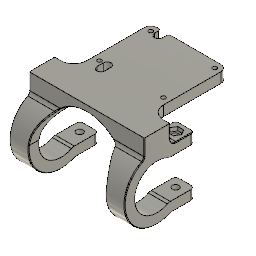
Screen Mount Assembly v8 (Autodesk Fusion 360 archive; units mm, degrees)
design "Mount"
Autodesk Fusion 360 part; units mm, degrees
note: some values were not read from the file. Set by a fixed rule: which face or edge a step refers to.
(part 1 of 2)
sketch "Sketch1" plane through (0, 0, -22.5) normal (0, 0, -1) x (1, 0, 0)
  circle A0 centre (-25, -20) radius 1.65
  circle A1 centre (25, 20) radius 1.65
  circle A2 centre (-25, 20) radius 1.65
  circle A3 centre (25, -20) radius 1.65
  circle A4 centre (25, 20) radius 5
  circle A5 centre (-25, 20) radius 5
  circle A6 centre (-25, -20) radius 5
  circle A7 centre (25, -20) radius 5
  line L0 (-25, -25) -> (25, -25)
  line L1 (30, -20) -> (30, 55)
  line L2 (30, 55) -> (-30, 55)
  line L3 (-30, 55) -> (-30, -20)
  line L4 (0, 0) -> (0, -45.9307) construction
  line L5 (0, 0) -> (62.0132, 0) construction
  dimension "d91" = 10
  dimension "d1" = 50
  dimension "d2" = 40
  dimension "d3" = 3.3
  dimension "d4" = 55
  constraint concentric A1 A4
  constraint concentric A2 A5
  constraint equal A4 A5
  constraint concentric A0 A6
  constraint concentric A3 A7
  constraint equal A4 A7
  constraint equal A4 A6
  constraint coincident A6 L0.start
  constraint coincident A7 L0.end
  constraint tangent A7 L0
  constraint tangent A6 L0
  constraint coincident A7 L1.start
  constraint tangent A7 L1
  constraint coincident A6 L3.end
  constraint tangent A6 L3
  constraint tangent A5 L3
  constraint tangent A4 L1
  constraint coincident L4.start L5.start
  constraint vertical L4
  constraint symmetric A0 A3 L4
  constraint symmetric A1 A2 L4
  constraint perpendicular L4 L5
  constraint symmetric A4 A7 L5
  constraint equal A1 A3
  constraint horizontal L2
  measures "d91" diameter of A4
  measures "d1" distance of A0.centre A3.centre
  measures "d2" distance of A1.centre A3.centre
  measures "d3" diameter of A3
  measures "d4" distance of L2 L5
extrude "Extrude1" add sketch "Sketch1" along normal blind 8 contours A4 | A5 | A6 A7 L0 L1 L2 L3 | A7 | A6
sketch "Sketch2" plane through (0, 0, -22.5) normal (0, 0, 1) x (-1, 0, 0)
  circle A0 centre (-25, -20) radius 1.65
  circle A1 centre (25, 20) radius 1.65
  circle A2 centre (25, -20) radius 1.65
  circle A3 centre (-25, 20) radius 1.65
  line L0 (30, -20) -> (30, 55)
  line L1 (30, 55) -> (-30, 55)
  line L2 (-30, 55) -> (-30, -20)
  arc A4 (-30, -20) -> (-25, -25) centre (-25, -20) ccw
  line L3 (-25, -25) -> (25, -25)
  arc A5 (25, -25) -> (30, -20) centre (25, -20) ccw
  line L4 (-30, 35) -> (-45, 35)
  line L5 (-45, 35) -> (-45, 55)
  line L6 (-45, 55) -> (-30, 55)
  line L7 (30, 55) -> (45, 55)
  line L8 (45, 55) -> (45, 35)
  line L9 (45, 35) -> (30, 35)
  line L10 (0, 55) -> (0, -10) construction
  dimension "d96" = 15
  dimension "d97" = 20
  constraint coincident L2 L4.start
  constraint perpendicular L2 L4
  constraint perpendicular L4 L5
  constraint coincident L1.end L2.start
  constraint perpendicular L2 L6
  constraint coincident L0.end L1.start
  constraint perpendicular L0 L7
  constraint perpendicular L7 L8
  constraint coincident L0 L9.end
  constraint perpendicular L0 L9
  constraint collinear L4 L9
  constraint midpoint L1 L10.start
  constraint perpendicular L1 L10
  constraint symmetric L5 L8 L10
  measures "d96" distance of L5.end L1.end
  measures "d97" distance of L4 L6
extrude "Extrude2" add sketch "Sketch2" against normal up to surface (8 mm away) contours L0 L7 L8 L9 | L2 L4 L5 L6
sketch "Sketch3" plane through (45, 0, 0) normal (1, 0, 0) x (0, 1, 0)
  line L0 (-55, -30.5) -> (-35, -30.5)
  line L1 (-35, -30.5) -> (-35, -22.5)
  line L2 (-35, -22.5) -> (-55, -22.5)
  line L3 (-55, -22.5) -> (-55, -30.5)
  circle A0 centre (-45, -60.5) radius 17.5
  circle A1 centre (-45, -60.5) radius 25.5
  line L4 (-35.9861, -45.5) -> (-15.5, -45.5)
  line L5 (-35.9861, -75.5) -> (-15.5, -75.5)
  line L6 (-27.5, -45.5) -> (-27.5, -75.5)
  line L7 (-45, -60.5) -> (22.9715, -60.5) construction
  line L8 (-55, -30.5) -> (-55, -37.0426)
  line L9 (-35, -30.5) -> (-35, -37.0426)
  line L10 (-45, -30.5) -> (-45, -60.5) construction
  line L11 (-33.9886, -37.5) -> (-15.5, -37.5)
  line L12 (-15.5, -37.5) -> (-15.5, -45.5)
  line L13 (-33.9886, -83.5) -> (-15.5, -83.5)
  line L14 (-15.5, -83.5) -> (-15.5, -75.5)
  dimension "d100" = 35
  dimension "d101" = 8
  dimension "d102" = 30
  dimension "d103" = 30
  dimension "d104" = 8
  dimension "d105" = 12
  constraint concentric A0 A1
  constraint coincident A0 L4.start
  constraint coincident A0 L5.start
  constraint horizontal L5
  constraint coincident L4 L6.start
  constraint coincident L5 L6.end
  constraint tangent A0 L6
  constraint vertical L6
  constraint coincident A0.centre A1.centre
  constraint horizontal L7
  constraint symmetric L4 L5 L7
  constraint coincident L0.start L3.end
  constraint coincident A1 L8.end
  constraint perpendicular L0 L8
  constraint coincident L0.end L1.start
  constraint coincident A1 L9.end
  constraint perpendicular L0 L9
  constraint midpoint L0 L10.start
  constraint perpendicular L0 L10
  constraint coincident A1 L11.start
  constraint parallel L4 L11
  constraint coincident A1 L13.start
  constraint perpendicular L12 L13
  constraint perpendicular L13 L14
  constraint collinear L12 L14
  constraint equal L12 L14
  measures "d100" diameter of A0 L7
  measures "d101" distance of A0 A1
  measures "d102" distance of L0 A0.centre
  measures "d103" distance of L4 L5
  measures "d104" distance of L4 L11
  measures "d105" distance of L6 L12
extrude "Extrude3" add sketch "Sketch3" against normal up to surface (90 mm away) contours L0 A1 L8 L9 | A0 A1 L4 L5 | A1 L5 L13 L14 | A1 L4 L11 L12
sketch "Sketch4" plane through (0, 0, -83.5) normal (0, 0, -1) x (1, 0, 0)
  circle A0 centre (37.5, 23) radius 2.65
  circle A1 centre (-37.5, 23) radius 2.65
  line L0 (0, 15.5) -> (0, 31.5) construction
  line L1 (-45, 33.9886) -> (-45, 15.5)
  line L2 (-45, 15.5) -> (45, 15.5)
  line L3 (45, 15.5) -> (45, 33.9886)
  line L4 (45, 33.9886) -> (-45, 33.9886)
  dimension "d109" = 5.3
  dimension "d25" = 7.5
  dimension "d26" = 7.5
  constraint symmetric A0 A1 L0
  constraint midpoint L0.start L2
  constraint perpendicular L0 L2
  measures "d109" diameter of A0
  measures "d25" distance of A0.centre L3
  measures "d26" distance of A0.centre L2
extrude "Extrude4" cut sketch "Sketch4" against normal up to surface (46 mm away) contours A0 | A1
sketch "Sketch7" plane through (0, 0, -37.5) normal (0, 0, 1) x (-1, 0, 0)
  circle A0 centre (-37.5, 23) radius 2.65
  circle A1 centre (37.5, 23) radius 2.65
  line L0 (45, 15.5) -> (45, 33.9886)
  line L1 (45, 33.9886) -> (-45, 33.9886)
  line L2 (-45, 33.9886) -> (-45, 15.5)
  line L3 (-45, 15.5) -> (45, 15.5)
  line L4 (35.1906, 27) -> (32.8812, 23)
  line L5 (32.8812, 23) -> (35.1906, 19)
  line L6 (35.1906, 19) -> (39.8094, 19)
  line L7 (39.8094, 19) -> (42.1188, 23)
  line L8 (42.1188, 23) -> (39.8094, 27)
  line L9 (39.8094, 27) -> (35.1906, 27)
  line L10 (-39.8094, 27) -> (-42.1188, 23)
  line L11 (-42.1188, 23) -> (-39.8094, 19)
  line L12 (-39.8094, 19) -> (-35.1906, 19)
  line L13 (-35.1906, 19) -> (-32.8812, 23)
  line L14 (-32.8812, 23) -> (-35.1906, 27)
  line L15 (-35.1906, 27) -> (-39.8094, 27)
  point P0 (37.5, 23)
  point P1 (-37.5, 23)
  dimension "d5" = 4
  constraint coincident P0 A1.centre
  constraint coincident A0.centre P1
  constraint horizontal L9
  constraint equal L9 L15
  constraint horizontal L15
  measures "d5" distance of P0 L9
extrude "Extrude5" cut sketch "Sketch7" against normal blind 3 contours L4 L5 L6 L7 L8 L9 | L10 L11 L12 L13 L14 L15
sketch "Sketch6" plane through (0, -55, 0) normal (0, -1, 0) x (1, 0, 0)
  line L0 (45, -22.5) -> (-45, -22.5)
  line L1 (-45, -22.5) -> (-45, -37.0426)
  line L2 (-45, -37.0426) -> (45, -37.0426)
  line L3 (45, -37.0426) -> (45, -22.5)
  line L4 (30, -30.5) -> (30, -91.7665)
  line L5 (45, -83.5) -> (45, -37.0426)
  line L6 (-30, -30.5) -> (-30, -95.0335)
  line L7 (-45, -80.5) -> (-45, -37.0426)
  line L8 (30, -30.5) -> (-30, -30.5)
  line L9 (-30, -30.5) -> (-25, -30.5)
  line L10 (-25, -30.5) -> (25, -30.5)
  line L11 (25, -30.5) -> (30, -30.5)
  line L12 (26.65, -30.5) -> (23.35, -30.5)
  line L13 (-23.35, -30.5) -> (-26.65, -30.5)
  line L14 (-23.35, -30.5) -> (-26.65, -30.5)
  line L15 (26.65, -30.5) -> (23.35, -30.5)
  arc A0 (30, -57.5) -> (-30, -57.5) centre (0, -57.5) ccw
  line L16 (40.15, -83.5) -> (34.85, -83.5)
  line L17 (-34.85, -83.5) -> (-40.15, -83.5)
  line L18 (-45, -83.5) -> (45, -83.5)
  line L19 (45, -83.5) -> (-45, -83.5)
  line L20 (-16.1649, -27.5) -> (17, -27.5) construction
  dimension "d31" = 3
  constraint coincident L2.end L3.start
  constraint coincident L1.end L2.start
  constraint perpendicular L2 L7
  constraint coincident L4.start L8.start
  constraint vertical L4
  constraint coincident L6.start L8.end
  constraint vertical L6
  constraint coincident L4 A0.start
  constraint tangent L6 A0
  constraint tangent L4 A0
  constraint coincident L6 A0.end
  constraint coincident L5.start L18.end
  constraint horizontal L20
  constraint tangent A0 L20
  measures "d31" distance of L8 L20
extrude "Extrude6" cut sketch "Sketch6" along normal blind 15.5 and the other way up to surface (39.5 mm away) contours L2 L4 L6 A0 L18 L19 | L2 L8 L10 A0 | L8 L10 A0
extrude "Extrude7" cut 1 faces at (-10, -41.3295, -83.5) along direction (0, 0, -1) blind 15
sketch "Sketch10" plane through (0, 0, -30.5) normal (0, 0, -1) x (1, 0, 0)
  line L0 (-13.0767, 35) -> (-30, 35)
  line L1 (-30, 35) -> (-30, -20)
  arc A0 (-30, -20) -> (-25, -25) centre (-25, -20) ccw
  line L2 (-25, -25) -> (25, -25)
  arc A1 (25, -25) -> (30, -20) centre (25, -20) ccw
  line L3 (30, -20) -> (30, 35)
  line L4 (30, 35) -> (13.0767, 35)
  circle A2 centre (-25, -20) radius 1.65
  circle A3 centre (25, 20) radius 1.65
  circle A4 centre (25, -20) radius 1.65
  circle A5 centre (-25, 20) radius 1.65
  line L5 (-13.0767, 15.5) -> (-13.0767, 35)
  line L6 (13.0767, 35) -> (13.0767, 15.5)
  line L7 (13.0767, 15.5) -> (-13.0767, 15.5)
extrude "Extrude9" cut sketch "Sketch10" along normal up to surface (53 mm away) contours L0 L1 A0 L2 A1 L3 L4 L5 L6 L7 | A2 | A3 | A4 | A5
fillet "Fillet1" radius 5 4 edges at (-37.5, -35.9861, -75.5) (37.5, -35.9861, -75.5) (-36.2477, -35.9861, -45.5) (36.2477, -35.9861, -45.5)
fillet "Fillet3" radius 5 4 edges at (37.5, -33.9886, -37.5) (-37.5, -33.9886, -37.5) (37.5, -35, -37.0426) (-37.5, -35, -37.0426)
fillet "Fillet3" radius 3 2 edges at (37.5, -33.9886, -83.5) (-37.5, -33.9886, -83.5)
fillet "Fillet3" radius 3 3 edges at (33.4715, -55, -37.0426) (-33.4715, -55, -37.0426) (33.4715, -55, -37.0426)
fillet "Fillet2" radius 5 2 edges at (-21.5383, -35, -30.5) (21.5383, -35, -30.5)
fillet "Fillet2" radius 10 2 edges at (-30, -35, -26.5) (30, -35, -26.5)
fillet "Fillet5" radius 3 6 edges at (-45, -15.5, -79.5) (-30, -15.5, -79.5) (45, -15.5, -79.5) (30, -15.5, -79.5) (45, -15.5, -41.5) (-45, -15.5, -41.5)
fillet "Fillet5" radius 3 2 edges at (-30, -15.5, -41.5) (30, -15.5, -41.5)
fillet "Fillet7" radius 2 4 edges at (-30, -35, -40.4953) (-30, -34.9421, -34.7412) (30, -34.9421, -34.7412) (30, -35, -40.4953)
fillet "Fillet8" radius 0.5 47 edges at (45, -55, -28.8188) (45, -55.4402, -36.702) (45, -67.9856, -71.5414) (45, -33.9557, -83.5665) (45, -25.9137, -83.5) (44.1213, -16.3787, -83.5) (37.5, -15.5, -83.5) (30.8787, -16.3787, -83.5) (30, -25.9137, -83.5) (30, -33.9557, -83.5665) (30, -60.0925, -81.054) (27.5466, -65.7069, -45.6182) (21.5129, -55.3759, -36.5909) (0, -55, -27.5) (-21.5129, -55.3759, -36.5909) (-27.5466, -65.7069, -45.6182) (-30, -60.0925, -81.054) (-30, -33.9557, -83.5665) (-30, -25.9137, -83.5) (-30.8787, -16.3787, -83.5) (-37.5, -15.5, -83.5) (-44.1213, -16.3787, -83.5) (-45, -25.9137, -83.5) (-45, -33.9557, -83.5665) (-45, -67.9856, -71.5414) (-45, -55.4402, -36.702) (-45, -55, -28.8188) (45, -35, -27.5) (45, -33.5355, -36.0355) (45, -24.25, -37.5) (44.1213, -16.3787, -37.5) (37.5, -15.5, -37.5) (30.8787, -16.3787, -37.5) (30, -24.25, -37.5) (30, -31.5811, -37.2434) (29.9254, -33.5435, -36.0277) (29.027, -34.6, -34.4596) (-45, -35, -27.5) (-45, -33.5355, -36.0355) (-45, -24.25, -37.5) (-44.1213, -16.3787, -37.5) (-37.5, -15.5, -37.5) (-30.8787, -16.3787, -37.5) (-30, -24.25, -37.5) (-30, -31.5811, -37.2434) (-29.9254, -33.5435, -36.0277) (-29.0637, -34.5848, -34.4949)
sketch "Sketch8" plane through (0, 0, -22.5) normal (0, 0, 1) x (-1, 0, 0)
  line L0 (-44.5, 35) -> (-40, 35)
  arc A0 (-30, 25) -> (-40, 35) centre (-40, 25) ccw
  line L1 (-30, 25) -> (-30, -20)
  arc A1 (-30, -20) -> (-25, -25) centre (-25, -20) ccw
  line L2 (-25, -25) -> (25, -25)
  arc A2 (25, -25) -> (30, -20) centre (25, -20) ccw
  line L3 (30, -20) -> (30, 25)
  arc A3 (40, 35) -> (30, 25) centre (40, 25) ccw
  line L4 (45, 35.5) -> (45, 54.5)
  line L5 (44.5, 55) -> (-44.5, 55)
  line L6 (-45, 54.5) -> (-45, 35.5)
  circle A4 centre (25, 20) radius 1.65
  circle A5 centre (-25, -20) radius 1.65
  circle A6 centre (-25, 20) radius 1.65
  circle A7 centre (25, -20) radius 1.65
  line L7 (16, -25) -> (16, -20)
  arc A8 (22, -20) -> (16, -20) centre (19, -20) ccw
  line L8 (22, -20) -> (22, -25)
  line L9 (16, 25) -> (16, 20)
  arc A9 (16, 20) -> (22, 20) centre (19, 20) ccw
  line L10 (22, 20) -> (22, 25)
  arc A10 (22, 25) -> (16, 25) centre (19, 25) ccw
  arc A11 (44.5, 35) -> (45, 35.5) centre (44.5, 35.5) ccw
  arc A12 (45, 54.5) -> (44.5, 55) centre (44.5, 54.5) ccw
  arc A13 (-44.5, 55) -> (-45, 54.5) centre (-44.5, 54.5) ccw
  arc A14 (-45, 35.5) -> (-44.5, 35) centre (-44.5, 35.5) ccw
  line L11 (40, 35) -> (44.5, 35)
  dimension "d9" = 3
  dimension "d10" = 5
  dimension "d23" = 3
  constraint coincident L2 L7.start
  constraint perpendicular L2 L7
  constraint tangent L7 A8
  constraint coincident L2 L8.end
  constraint tangent A8 L8
  constraint perpendicular L2 L8
  constraint horizontal A1.centre A8.centre
  constraint vertical L9
  constraint tangent L9 A9
  constraint tangent A9 L10
  constraint parallel L9 L10
  constraint tangent L10 A10
  constraint equal A8 A9
  constraint tangent L9 A10
  constraint horizontal A6.centre A9.centre
  constraint vertical A8.centre A9.centre
  measures "d9" radius of A8
  measures "d10" distance of A9.centre A10.centre
  measures "d23" distance of A2.centre L8
extrude "Extrude8" cut sketch "Sketch8" against normal up to surface (8 mm away) contours L2 L7 A8 L8 | L9 A9 L10 A10
fillet "Fillet6" radius 2 2 edges at (-16, 25, -26.5) (-22, 25, -26.5)
fillet "Fillet9" radius 2 2 edges at (0, -15.5, -27.5) (0, -15.5, -30.5)
fillet "Fillet10" radius 1 8 edges at (24.4592, -35, -40.1291) (16.1121, -33.7515, -32.1946) (13.0767, -22.3745, -30.5) (12.9586, -14.0545, -30.5) (-12.9598, -14.058, -30.5) (-13.0767, -22.3745, -30.5) (-16.1121, -33.7515, -32.1946) (-24.4592, -35, -40.1291)

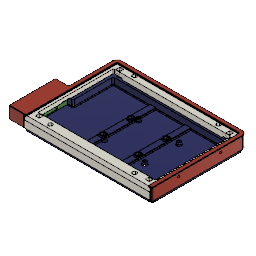
design "7inch Screen Mount"
Autodesk Fusion 360 part; units mm, degrees
sketch "Sketch1" plane through (0, 0, 0) normal (0, 0, 1) x (1, 0, 0) in component "Main Body"
  line L0 (83.75, -54) -> (-83.75, -54)
  line L1 (-83.75, -54) -> (-83.75, 54)
  line L2 (-83.75, 54) -> (83.75, 54)
  line L3 (83.75, 54) -> (83.75, -54)
  line L4 (83.75, -54) -> (-83.75, 54) construction
  line L5 (-83.75, -54) -> (83.75, 54) construction
  line L6 (90, 65) -> (-90, 65)
  line L7 (-90, 65) -> (-90, -65)
  line L8 (-90, -65) -> (90, -65)
  line L9 (90, -65) -> (90, 65)
  line L10 (90, 65) -> (-90, -65) construction
  line L11 (-90, 65) -> (90, -65) construction
  dimension "d1_1" = 167.5
  dimension "d2_1" = 108
  dimension "d3_1" = 180
  dimension "d4_1" = 130
  constraint horizontal L0
  constraint perpendicular L0 L1
  constraint parallel L0 L2
  constraint parallel L1 L3
  constraint coincident L4 origin
  constraint coincident L5 origin
  constraint horizontal L6
  constraint perpendicular L6 L7
  constraint parallel L6 L8
  constraint parallel L7 L9
  constraint coincident L10 origin
  constraint coincident L11 origin
  measures "d1_1" distance of L1.end L2.end
  measures "d2_1" distance of L0.end L1.end
  measures "d3_1" distance of L7.end L8.end
  measures "d4_1" distance of L6.end L7.end
extrude "Extrude1" add sketch "Sketch1" against normal blind 5.8 makes body 1 in component "Main Body"
sketch "Sketch3" plane through (0, 0, -5.8) normal (0, 0, -1) x (1, 0, 0) in component "Main Body"
  line L0 (83.75, -54) -> (-83.75, -54)
  line L1 (-83.75, -54) -> (-83.75, 54)
  line L2 (-83.75, 54) -> (83.75, 54)
  line L3 (83.75, 54) -> (83.75, -54)
  line L4 (90, -65) -> (90, 65)
  line L5 (90, 65) -> (-90, 65)
  line L6 (-90, 65) -> (-90, -65)
  line L7 (-90, -65) -> (90, -65)
  line L8 (88, 63) -> (-88, 63)
  line L9 (88, -63) -> (-88, -63)
  line L10 (0, 0) -> (55, 0) construction
  line L11 (0, 0) -> (0, 36.0005) construction
  circle A0 centre (78.5, 57.5) radius 1.65
  circle A1 centre (78.5, -57.5) radius 1.65
  circle A2 centre (-78.5, -57.5) radius 1.65
  circle A3 centre (-78.5, 57.5) radius 1.65
  line L12 (88, -63) -> (88, 63)
  line L13 (-88, -63) -> (-88, 63)
  line L14 (-73.75, 63) -> (-73.75, 54)
  line L15 (73.75, 63) -> (73.75, 54)
  line L16 (73.75, -54) -> (73.75, -63)
  line L17 (-73.75, -54) -> (-73.75, -63)
  dimension "d19_1" = 157
  dimension "d20_1" = 115
  dimension "d21_1" = 3.3
  dimension "d83_1" = 2
  dimension "d1" = 2
  dimension "d2" = 10
  constraint coincident L10.start L11.start
  constraint perpendicular L3 L10
  constraint symmetric L8 L9 L10
  constraint perpendicular L10 L11
  constraint symmetric L11 A0 A3
  constraint symmetric L11 A1 A2
  constraint symmetric L10 A0 A1
  constraint perpendicular L2 L12
  constraint coincident L8.start L12.end
  constraint symmetric L11 L12 L13
  constraint coincident L8 L14.start
  constraint coincident L2 L14.end
  constraint perpendicular L2 L14
  constraint coincident L8 L15.start
  constraint coincident L2 L15.end
  constraint perpendicular L2 L15
  constraint coincident L9 L16.end
  constraint perpendicular L9 L16
  constraint coincident L0 L17.start
  constraint coincident L9 L17.end
  constraint perpendicular L9 L17
  constraint symmetric L11 L14 L15
  constraint collinear L15 L16
  constraint collinear L14 L17
  constraint coincident L0 L16.start
  measures "d19_1" distance of A0.centre A3.centre
  measures "d20_1" vertical distance of A0.centre A1.centre
  measures "d21_1" diameter of A3
  measures "d83_1" distance of L4 L12
  measures "d1" distance of L5 L8
  measures "d2" distance of L1 L14
extrude "Extrude3" add sketch "Sketch3" along normal blind 2 contours L0 L9 L16 L17 | L2 L8 L14 L15 | L4 L5 L6 L7 bodies 1 in component "Main Body"
extrude "Extrude4" cut sketch "Sketch3" against normal up to surface (5.8 mm away) contours A0 | A1 | A2 | A3 bodies 1 in component "Main Body"
sketch "Sketch5" plane through (0, 0, -7.8) normal (0, 0, -1) x (1, 0, 0) in component "Main Body"
  line L0 (-90, -65) -> (90, -65)
  line L1 (90, -65) -> (90, 65)
  line L2 (90, 65) -> (-90, 65)
  line L3 (-90, 65) -> (-90, -65)
  line L4 (-83.75, 54) -> (83.75, 54)
  line L5 (83.75, 54) -> (73.75, 54)
  line L6 (-73.75, -63) -> (-88, -63)
  line L7 (-88, 63) -> (-73.75, 63)
  line L8 (88, 63) -> (88, -63)
  line L9 (-88, -63) -> (-88, 63)
  line L10 (-88, 54) -> (-90, 54)
  line L11 (-90, 4) -> (-88, 4)
  line L12 (73.75, -63) -> (73.75, -54)
  line L13 (73.75, -54) -> (-73.75, -54)
  line L14 (-73.75, -54) -> (-73.75, -63)
  line L15 (-73.75, 63) -> (-73.75, 54)
  line L16 (-73.75, 54) -> (73.75, 54)
  line L17 (73.75, 54) -> (73.75, 63)
  line L18 (73.75, 63) -> (88, 63)
  line L19 (88, -63) -> (73.75, -63)
  line L20 (73.75, 54) -> (-73.75, 54)
  line L21 (-73.75, 54) -> (-83.75, 54)
  line L22 (83.75, -54) -> (73.75, -54)
  line L23 (-73.75, -54) -> (-83.75, -54)
  dimension "d59" = 50
  constraint coincident L9 L10.start
  constraint coincident L3 L10.end
  constraint perpendicular L3 L10
  constraint collinear L5 L10
  constraint coincident L3 L11.start
  constraint coincident L9 L11.end
  constraint perpendicular L9 L11
  measures "d59" distance of L10 L11
extrude "Extrude6" cut sketch "Sketch5" against normal up to surface (2 mm away) contours L3 L9 L10 L11 bodies 1 in component "Main Body"
sketch "Sketch13" plane through (0, 0, -5.8) normal (0, 0, -1) x (1, 0, 0) in component "Main Body"
  circle A0 centre (-78.5, -57.5) radius 1.65
  circle A1 centre (-78.5, 57.5) radius 1.65
  line L0 (-73.75, 54) -> (-73.75, 63)
  line L1 (-73.75, 63) -> (-88, 63)
  line L2 (-88, 63) -> (-88, 54)
  line L3 (-88, 54) -> (-90, 54)
  line L4 (-90, 54) -> (-90, 4)
  line L5 (-90, 4) -> (-88, 4)
  line L6 (-88, 4) -> (-88, -63)
  line L7 (-88, -63) -> (-73.75, -63)
  line L8 (-73.75, -63) -> (-73.75, -54)
  line L9 (-73.75, -54) -> (-83.75, -54)
  line L10 (-83.75, -54) -> (-83.75, 54)
  line L11 (-83.75, 54) -> (-73.75, 54)
  line L12 (-90, 19) -> (-83.75, 19)
  line L13 (-90, 9) -> (-83.75, 9)
  dimension "d127" = 35
  dimension "d128" = 10
  constraint coincident L4 L12.start
  constraint coincident L10 L12.end
  constraint perpendicular L10 L12
  constraint coincident L4 L13.start
  constraint coincident L10 L13.end
  constraint perpendicular L10 L13
  measures "d127" distance of L11 L12
  measures "d128" distance of L12 L13
extrude "Extrude14" cut sketch "Sketch13" against normal blind 1 contours L4 L10 L12 L13 bodies 1 in component "Main Body"
fillet "Fillet11" radius 0.5 4 edges at (-86.875, -19, -4.8) (-86.875, -19, -5.8) (-86.875, -9, -4.8) (-86.875, -9, -5.8) on bodies 1 in component "Main Body"
sketch "Sketch4" plane through (0, 0, 0) normal (0, 0, 1) x (-1, 0, 0) in component "Main Body"
  circle A0 centre (-78.5, -57.5) radius 1.65
  circle A1 centre (-78.5, 57.5) radius 1.65
  circle A2 centre (78.5, -57.5) radius 1.65
  circle A3 centre (78.5, 57.5) radius 1.65
  line L0 (83.75, -54) -> (-83.75, -54)
  line L1 (-83.75, -54) -> (-83.75, 54)
  line L2 (-83.75, 54) -> (83.75, 54)
  line L3 (83.75, 54) -> (83.75, -54)
  line L4 (-81.225, -54.775) -> (-75.775, -54.775)
  line L5 (-75.775, -54.775) -> (-75.775, -60.225)
  line L6 (-75.775, -60.225) -> (-81.225, -60.225)
  line L7 (-81.225, -60.225) -> (-81.225, -54.775)
  line L8 (-81.225, -54.775) -> (-75.775, -60.225) construction
  line L9 (-75.775, -54.775) -> (-81.225, -60.225) construction
  line L10 (75.775, -54.775) -> (81.225, -54.775)
  line L11 (81.225, -54.775) -> (81.225, -60.225)
  line L12 (81.225, -60.225) -> (75.775, -60.225)
  line L13 (75.775, -60.225) -> (75.775, -54.775)
  line L14 (75.775, -54.775) -> (81.225, -60.225) construction
  line L15 (81.225, -54.775) -> (75.775, -60.225) construction
  line L16 (75.775, 54.775) -> (81.225, 54.775)
  line L17 (81.225, 54.775) -> (81.225, 60.225)
  line L18 (81.225, 60.225) -> (75.775, 60.225)
  line L19 (75.775, 60.225) -> (75.775, 54.775)
  line L20 (75.775, 54.775) -> (81.225, 60.225) construction
  line L21 (81.225, 54.775) -> (75.775, 60.225) construction
  line L22 (-75.775, 54.775) -> (-81.225, 54.775)
  line L23 (-81.225, 54.775) -> (-81.225, 60.225)
  line L24 (-81.225, 60.225) -> (-75.775, 60.225)
  line L25 (-75.775, 60.225) -> (-75.775, 54.775)
  line L26 (-75.775, 54.775) -> (-81.225, 60.225) construction
  line L27 (-81.225, 54.775) -> (-75.775, 60.225) construction
  line L28 (-90, 65) -> (-90, -65)
  line L29 (-90, -65) -> (90, -65)
  line L30 (90, -65) -> (90, 65)
  line L31 (90, 65) -> (-90, 65)
  point P0 (-78.5, -57.5)
  point P1 (78.5, -57.5)
  point P2 (78.5, 57.5)
  point P3 (-78.5, 57.5)
  dimension "d28_1" = 5.45
  constraint horizontal L4
  constraint perpendicular L4 L5
  constraint parallel L4 L6
  constraint parallel L5 L7
  constraint coincident L8 P0
  constraint coincident L9 P0
  constraint coincident P0 A0.centre
  constraint equal L5 L6
  constraint horizontal L10
  constraint perpendicular L10 L11
  constraint parallel L10 L12
  constraint parallel L11 L13
  constraint coincident L14 P1
  constraint coincident L15 P1
  constraint coincident P1 A2.centre
  constraint horizontal L16
  constraint perpendicular L16 L17
  constraint parallel L16 L18
  constraint parallel L17 L19
  constraint coincident L20 P2
  constraint coincident L21 P2
  constraint coincident P2 A3.centre
  constraint horizontal L22
  constraint perpendicular L22 L23
  constraint parallel L22 L24
  constraint parallel L23 L25
  constraint coincident L26 P3
  constraint coincident L27 P3
  constraint coincident P3 A1.centre
  constraint equal L5 L13
  constraint equal L6 L12
  constraint equal L6 L24
  constraint equal L5 L25
  constraint equal L12 L18
  constraint equal L13 L19
  measures "d28_1" distance of L4.end L5.end
extrude "Extrude5" cut sketch "Sketch4" against normal blind 4 contours L4 L5 L6 L7 | L10 L11 L12 L13 | L16 L17 L18 L19 | L22 L23 L24 L25 bodies 1 in component "Main Body"
sketch "Sketch12" plane through (-90, 0, 0) normal (-1, 0, 0) x (0, -1, 0) in component "Main Body"
  line L0 (54, -5.8) -> (54, -7.8)
  line L1 (54, -7.8) -> (65, -7.8)
  line L2 (65, -7.8) -> (65, 0)
  line L3 (65, 0) -> (-65, 0)
  line L4 (-65, 0) -> (-65, -7.8)
  line L5 (-65, -7.8) -> (4, -7.8)
  line L6 (4, -7.8) -> (4, -5.8)
  line L7 (19.5, -5.8) -> (54, -5.8)
  circle A0 centre (30, -3) radius 1.425
  line L8 (0, 0) -> (0, 35) construction
  circle A1 centre (-30, -3) radius 1.425
  arc A2 (8.5, -5.8) -> (9, -5.3) centre (8.5, -5.3) ccw
  arc A3 (9.5, -4.8) -> (9, -5.3) centre (9.5, -5.3) ccw
  line L9 (9.5, -4.8) -> (18.5, -4.8)
  arc A4 (19, -5.3) -> (18.5, -4.8) centre (18.5, -5.3) ccw
  arc A5 (19, -5.3) -> (19.5, -5.8) centre (19.5, -5.3) ccw
  line L10 (4, -5.8) -> (8.5, -5.8)
  dimension "d66" = 30
  dimension "d67" = 2.85
  dimension "d68" = 3
  constraint coincident L8.start origin
  constraint perpendicular L3 L8
  constraint symmetric A0 L8 A1
  measures "d66" horizontal distance of L8.start A0.centre
  measures "d67" diameter of A0
  measures "d68" distance of L3 A0.centre
extrude "Extrude7" cut sketch "Sketch12" against normal up to surface (180 mm away) contours A0 | A1 bodies 1 in component "Main Body"
sketch "Sketch8" plane through (0, 65, 0) normal (0, 1, 0) x (-1, 0, 0) in component "Main Body"
  line L0 (90, 0) -> (-90, 0)
  line L1 (-90, 0) -> (-90, -7.8)
  line L2 (-90, -7.8) -> (90, -7.8)
  line L3 (90, -7.8) -> (90, 0)
  line L4 (0, 0) -> (0, 45) construction
  circle A0 centre (70, -4) radius 1.425
  line L5 (80.15, -5.8) -> (76.85, -5.8)
  line L6 (78.5, -5.8) -> (78.5, 7.2) construction
  circle A1 centre (0, -4) radius 1.425
  circle A2 centre (-70, -4) radius 1.425
  dimension "d27" = 2.85
  dimension "d28" = 4
  dimension "d29" = 70
  dimension "d30" = 8.5
  dimension "d33" = -70
  dimension "d34" = 0
  constraint coincident L4.start origin
  constraint perpendicular L0 L4
  constraint midpoint L5 L6.start
  constraint perpendicular L5 L6
  measures "d27" diameter of A0
  measures "d28" distance of L0 A0.centre
  measures "d29" distance of L4 A0.centre
  measures "d30" distance of A0.centre L6
extrude "Extrude10" cut sketch "Sketch8" against normal up to surface (10 mm away) contours A0 | A1 | A2 bodies 1 in component "Main Body"
sketch "Sketch9" plane through (-83.75, 0, 0) normal (1, 0, 0) x (0, 1, 0) in component "Main Body"
  line L0 (54, 0) -> (-54, 0)
  line L1 (-54, 0) -> (-54, -5.8)
  line L2 (-8.5, -5.8) -> (54, -5.8)
  line L3 (54, -5.8) -> (54, 0)
  circle A0 centre (-30, -3) radius 1.425
  circle A1 centre (30, -3) radius 1.425
  arc A2 (-9, -5.3) -> (-8.5, -5.8) centre (-8.5, -5.3) ccw
  line L4 (-54, -5.8) -> (-19.5, -5.8)
  arc A3 (-19.5, -5.8) -> (-19, -5.3) centre (-19.5, -5.3) ccw
  arc A4 (-18.5, -4.8) -> (-19, -5.3) centre (-18.5, -5.3) ccw
  line L5 (-18.5, -4.8) -> (-9.5, -4.8)
  arc A5 (-9, -5.3) -> (-9.5, -4.8) centre (-9.5, -5.3) ccw
extrude "Extrude11" add sketch "Sketch9" against normal blind 1 contours A0 | A1 bodies 1 in component "Main Body"
sketch "Sketch10" plane through (83.75, 0, 0) normal (-1, 0, 0) x (0, -1, 0) in component "Main Body"
  line L0 (54, 0) -> (-54, 0)
  line L1 (-54, 0) -> (-54, -5.8)
  line L2 (-54, -5.8) -> (54, -5.8)
  line L3 (54, -5.8) -> (54, 0)
  circle A0 centre (30, -3) radius 1.425
  circle A1 centre (-30, -3) radius 1.425
extrude "Extrude12" add sketch "Sketch10" against normal blind 1 contours A0 | A1 bodies 1 in component "Main Body"
fillet "Fillet7" radius 4 2 edges at (90, 65, -3.9) (-90, 65, -3.9) on bodies 1 in component "Main Body"
fillet "Fillet8" radius 2 12 edges at (88, -63, -6.8) (73.75, -63, -6.8) (73.75, -54, -6.8) (73.75, 63, -6.8) (73.75, 54, -6.8) (88, 63, -6.8) (-73.75, 54, -6.8) (-73.75, 63, -6.8) (-88, 63, -6.8) (-73.75, -63, -6.8) (-73.75, -54, -6.8) (-88, -63, -6.8) on bodies 1 in component "Main Body"
fillet "Fillet9" radius 1 4 edges at (-83.75, -54, -2.9) (-83.75, 54, -2.9) (83.75, 54, -2.9) (83.75, -54, -2.9) on bodies 1 in component "Main Body"
sketch "Sketch6" plane through (0, 0, -7.8) normal (0, 0, -1) x (1, 0, 0) in component "Main Body"
  arc A0 (-73.75, 56) -> (-71.75, 54) centre (-71.75, 56) ccw
  line L0 (-71.75, 54) -> (71.75, 54)
  arc A1 (71.75, 54) -> (73.75, 56) centre (71.75, 56) ccw
  line L1 (73.75, 56) -> (73.75, 61)
  arc A2 (75.75, 63) -> (73.75, 61) centre (75.75, 61) ccw
  line L2 (75.75, 63) -> (86, 63)
  arc A3 (88, 61) -> (86, 63) centre (86, 61) ccw
  line L3 (88, 61) -> (88, -61)
  arc A4 (86, -63) -> (88, -61) centre (86, -61) ccw
  line L4 (86, -63) -> (75.75, -63)
  arc A5 (73.75, -61) -> (75.75, -63) centre (75.75, -61) ccw
  line L5 (73.75, -61) -> (73.75, -56)
  arc A6 (73.75, -56) -> (71.75, -54) centre (71.75, -56) ccw
  line L6 (71.75, -54) -> (-71.75, -54)
  arc A7 (-71.75, -54) -> (-73.75, -56) centre (-71.75, -56) ccw
  line L7 (-73.75, -56) -> (-73.75, -61)
  arc A8 (-75.75, -63) -> (-73.75, -61) centre (-75.75, -61) ccw
  line L8 (-75.75, -63) -> (-86, -63)
  arc A9 (-88, -61) -> (-86, -63) centre (-86, -61) ccw
  line L9 (-88, -61) -> (-88, 4)
  line L10 (-88, 4) -> (-90, 4)
  line L11 (-90, 4) -> (-90, -61)
  arc A10 (-90, -61) -> (-86, -65) centre (-86, -61) ccw
  line L12 (-86, -65) -> (86, -65)
  arc A11 (86, -65) -> (90, -61) centre (86, -61) ccw
  line L13 (90, -61) -> (90, 65)
  line L14 (90, 65) -> (-90, 65)
  line L15 (-90, 54) -> (-88, 54)
  line L16 (-88, 54) -> (-88, 61)
  arc A12 (-86, 63) -> (-88, 61) centre (-86, 61) ccw
  line L17 (-86, 63) -> (-75.75, 63)
  arc A13 (-73.75, 61) -> (-75.75, 63) centre (-75.75, 61) ccw
  line L18 (-73.75, 61) -> (-73.75, 56)
  line L19 (0, 0) -> (0, 82.8425) construction
  line L20 (0, 0) -> (120, 0) construction
  circle A14 centre (60, 60) radius 1.65
  circle A15 centre (-60, 60) radius 1.65
  circle A16 centre (60, -60) radius 1.65
  circle A17 centre (-60, -60) radius 1.65
  line L21 (-90, 65) -> (-90, 54)
  dimension "d17" = 60
  dimension "d18" = 3.3
  dimension "d19" = 60
  constraint coincident L19.start L20.start
  constraint perpendicular L14 L19
  constraint horizontal L20
  constraint symmetric L19 A14 A15
  constraint symmetric L20 A14 A16
  constraint symmetric L20 A15 A17
  measures "d17" distance of L20 A14.centre
  measures "d18" diameter of A14
  measures "d19" distance of L19 A14.centre
extrude "Extrude8" cut sketch "Sketch6" against normal up to surface (7.8 mm away) contours A14 | A15 | A16 | A17 bodies 1 in component "Main Body"
sketch "Sketch7" plane through (0, 0, 0) normal (0, 0, 1) x (-1, 0, 0) in component "Main Body"
  circle A0 centre (-60, 60) radius 1.65
  circle A1 centre (-60, -60) radius 1.65
  circle A2 centre (60, 60) radius 1.65
  circle A3 centre (60, -60) radius 1.65
  arc A4 (86, -65) -> (90, -61) centre (86, -61) ccw
  line L0 (90, -61) -> (90, 65)
  line L1 (90, 65) -> (-90, 65)
  line L2 (-90, 65) -> (-90, -61)
  arc A5 (-90, -61) -> (-86, -65) centre (-86, -61) ccw
  line L3 (-86, -65) -> (86, -65)
  line L4 (-81.225, 54.775) -> (-81.225, 60.225)
  line L5 (-81.225, 60.225) -> (-75.775, 60.225)
  line L6 (-75.775, 60.225) -> (-75.775, 54.775)
  line L7 (-75.775, 54.775) -> (-81.225, 54.775)
  line L8 (-75.775, -54.775) -> (-75.775, -60.225)
  line L9 (-75.775, -60.225) -> (-81.225, -60.225)
  line L10 (-81.225, -60.225) -> (-81.225, -54.775)
  line L11 (-81.225, -54.775) -> (-75.775, -54.775)
  line L12 (81.225, 54.775) -> (75.775, 54.775)
  line L13 (75.775, 54.775) -> (75.775, 60.225)
  line L14 (75.775, 60.225) -> (81.225, 60.225)
  line L15 (81.225, 60.225) -> (81.225, 54.775)
  line L16 (81.225, -54.775) -> (81.225, -60.225)
  line L17 (81.225, -60.225) -> (75.775, -60.225)
  line L18 (75.775, -60.225) -> (75.775, -54.775)
  line L19 (75.775, -54.775) -> (81.225, -54.775)
  line L20 (82.75, -54) -> (-82.75, -54)
  arc A6 (-83.75, -53) -> (-82.75, -54) centre (-82.75, -53) ccw
  line L21 (-83.75, -53) -> (-83.75, 53)
  arc A7 (-82.75, 54) -> (-83.75, 53) centre (-82.75, 53) ccw
  line L22 (-82.75, 54) -> (82.75, 54)
  arc A8 (83.75, 53) -> (82.75, 54) centre (82.75, 53) ccw
  line L23 (83.75, 53) -> (83.75, -53)
  arc A9 (82.75, -54) -> (83.75, -53) centre (82.75, -53) ccw
  line L24 (-61.5877, -57.25) -> (-63.1754, -60)
  line L25 (-63.1754, -60) -> (-61.5877, -62.75)
  line L26 (-61.5877, -62.75) -> (-58.4123, -62.75)
  line L27 (-58.4123, -62.75) -> (-56.8246, -60)
  line L28 (-56.8246, -60) -> (-58.4123, -57.25)
  line L29 (-58.4123, -57.25) -> (-61.5877, -57.25)
  line L30 (58.4123, -57.25) -> (56.8246, -60)
  line L31 (56.8246, -60) -> (58.4123, -62.75)
  line L32 (58.4123, -62.75) -> (61.5877, -62.75)
  line L33 (61.5877, -62.75) -> (63.1754, -60)
  line L34 (63.1754, -60) -> (61.5877, -57.25)
  line L35 (61.5877, -57.25) -> (58.4123, -57.25)
  line L36 (61.5877, 57.25) -> (63.1754, 60)
  line L37 (63.1754, 60) -> (61.5877, 62.75)
  line L38 (61.5877, 62.75) -> (58.4123, 62.75)
  line L39 (58.4123, 62.75) -> (56.8246, 60)
  line L40 (56.8246, 60) -> (58.4123, 57.25)
  line L41 (58.4123, 57.25) -> (61.5877, 57.25)
  line L42 (-58.4123, 57.25) -> (-56.8246, 60)
  line L43 (-56.8246, 60) -> (-58.4123, 62.75)
  line L44 (-58.4123, 62.75) -> (-61.5877, 62.75)
  line L45 (-61.5877, 62.75) -> (-63.1754, 60)
  line L46 (-63.1754, 60) -> (-61.5877, 57.25)
  line L47 (-61.5877, 57.25) -> (-58.4123, 57.25)
  point P0 (-60, -60)
  point P1 (60, -60)
  point P2 (60, 60)
  point P3 (-60, 60)
  dimension "d22" = 2.75
  constraint coincident P0 A1.centre
  constraint horizontal L29
  constraint coincident P1 A3.centre
  constraint coincident P2 A2.centre
  constraint coincident P3 A0.centre
  constraint equal L35 L41
  constraint equal L41 L47
  constraint equal L29 L47
  constraint horizontal L35
  constraint horizontal L41
  constraint horizontal L47
  measures "d22" distance of P0 L29
extrude "Extrude9" cut sketch "Sketch7" against normal blind 5 contours L24 L25 L26 L27 L28 L29 | L30 L31 L32 L33 L34 L35 | L36 L37 L38 L39 L40 L41 | L42 L43 L44 L45 L46 L47 bodies 1 in component "Main Body"
sketch "Sketch11" plane through (0, 0, 0) normal (0, 0, 1) x (-1, 0, 0) in component "Main Body"
  line L0 (-63.1754, -60) -> (-61.5877, -57.25)
  line L1 (-61.5877, -57.25) -> (-58.4123, -57.25)
  line L2 (-58.4123, -57.25) -> (-56.8246, -60)
  line L3 (-56.8246, -60) -> (-58.4123, -62.75)
  line L4 (-58.4123, -62.75) -> (-61.5877, -62.75)
  line L5 (-61.5877, -62.75) -> (-63.1754, -60)
  line L6 (-56.8246, 60) -> (-58.4123, 57.25)
  line L7 (-58.4123, 57.25) -> (-61.5877, 57.25)
  line L8 (-61.5877, 57.25) -> (-63.1754, 60)
  line L9 (-63.1754, 60) -> (-61.5877, 62.75)
  line L10 (-61.5877, 62.75) -> (-58.4123, 62.75)
  line L11 (-58.4123, 62.75) -> (-56.8246, 60)
  line L12 (56.8246, -60) -> (58.4123, -57.25)
  line L13 (58.4123, -57.25) -> (61.5877, -57.25)
  line L14 (61.5877, -57.25) -> (63.1754, -60)
  line L15 (63.1754, -60) -> (61.5877, -62.75)
  line L16 (61.5877, -62.75) -> (58.4123, -62.75)
  line L17 (58.4123, -62.75) -> (56.8246, -60)
  line L18 (63.1754, 60) -> (61.5877, 57.25)
  line L19 (61.5877, 57.25) -> (58.4123, 57.25)
  line L20 (58.4123, 57.25) -> (56.8246, 60)
  line L21 (56.8246, 60) -> (58.4123, 62.75)
  line L22 (58.4123, 62.75) -> (61.5877, 62.75)
  line L23 (61.5877, 62.75) -> (63.1754, 60)
  arc A0 (86, -65) -> (90, -61) centre (86, -61) ccw
  line L24 (90, -61) -> (90, 65)
  line L25 (90, 65) -> (-90, 65)
  line L26 (-90, 65) -> (-90, -61)
  arc A1 (-90, -61) -> (-86, -65) centre (-86, -61) ccw
  line L27 (-86, -65) -> (86, -65)
  line L28 (-81.225, 54.775) -> (-81.225, 60.225)
  line L29 (-81.225, 60.225) -> (-75.775, 60.225)
  line L30 (-75.775, 60.225) -> (-75.775, 54.775)
  line L31 (-75.775, 54.775) -> (-81.225, 54.775)
  line L32 (-75.775, -54.775) -> (-75.775, -60.225)
  line L33 (-75.775, -60.225) -> (-81.225, -60.225)
  line L34 (-81.225, -60.225) -> (-81.225, -54.775)
  line L35 (-81.225, -54.775) -> (-75.775, -54.775)
  line L36 (81.225, 54.775) -> (75.775, 54.775)
  line L37 (75.775, 54.775) -> (75.775, 60.225)
  line L38 (75.775, 60.225) -> (81.225, 60.225)
  line L39 (81.225, 60.225) -> (81.225, 54.775)
  line L40 (81.225, -54.775) -> (81.225, -60.225)
  line L41 (81.225, -60.225) -> (75.775, -60.225)
  line L42 (75.775, -60.225) -> (75.775, -54.775)
  line L43 (75.775, -54.775) -> (81.225, -54.775)
  line L44 (82.75, -54) -> (-82.75, -54)
  arc A2 (-83.75, -53) -> (-82.75, -54) centre (-82.75, -53) ccw
  line L45 (-83.75, -53) -> (-83.75, 53)
  arc A3 (-82.75, 54) -> (-83.75, 53) centre (-82.75, 53) ccw
  line L46 (-82.75, 54) -> (82.75, 54)
  arc A4 (83.75, 53) -> (82.75, 54) centre (82.75, 53) ccw
  line L47 (83.75, 53) -> (83.75, -53)
  arc A5 (82.75, -54) -> (83.75, -53) centre (82.75, -53) ccw
  line L48 (-90, 65) -> (-90, 68)
  line L49 (-90, 68) -> (90, 68)
  line L50 (90, 68) -> (90, 65)
  dimension "d41" = 3
  constraint coincident L25.end L26.start
  constraint perpendicular L25 L48
  constraint perpendicular L48 L49
  constraint perpendicular L49 L50
  constraint coincident L24.end L25.start
  measures "d41" distance of L25.end L48.end
extrude "Extrude13" add sketch "Sketch11" against normal blind 15 contours L25 L48 L49 L50 bodies 1 in component "Main Body"
chamfer "Chamfer1" distance 5 distance2 2 1 edges at (0, -68, 0) measured on face at (30, -68, -10) on bodies 1 in component "Main Body"
fillet "Fillet10" radius 0.5 4 edges at (90, -68, -10) (90, -67, -2.5) (-90, -68, -10) (-90, -67, -2.5) on bodies 1 in component "Main Body"
sketch "Sketch1 (2)" plane through (0, 0, 0) normal (0, 0, 1) x (-1, 0, 0) in component "Top Cover"
  ellipse E0 centre (89.5, 65.4615) end of major axis (89.5, 66) minor radius 0.5 (90, 65.4615) -> (89.5, 66) ccw
  line L0 (89.5, 66) -> (-89.5, 66)
  ellipse E1 centre (-89.5, 65.4615) end of major axis (-89.5, 66) minor radius 0.5 (-89.5, 66) -> (-90, 65.4615) ccw
  line L1 (-90, 65.4615) -> (-90, -61)
  arc A0 (-90, -61) -> (-86, -65) centre (-86, -61) ccw
  line L2 (-86, -65) -> (86, -65)
  arc A1 (86, -65) -> (90, -61) centre (86, -61) ccw
  line L3 (90, -61) -> (90, 65.4615)
  line L4 (-63.1754, -60) -> (-61.5877, -57.25)
  line L5 (-61.5877, -57.25) -> (-58.4123, -57.25)
  line L6 (-58.4123, -57.25) -> (-56.8246, -60)
  line L7 (-56.8246, -60) -> (-58.4123, -62.75)
  line L8 (-58.4123, -62.75) -> (-61.5877, -62.75)
  line L9 (-61.5877, -62.75) -> (-63.1754, -60)
  line L10 (-56.8246, 60) -> (-58.4123, 57.25)
  line L11 (-58.4123, 57.25) -> (-61.5877, 57.25)
  line L12 (-61.5877, 57.25) -> (-63.1754, 60)
  line L13 (-63.1754, 60) -> (-61.5877, 62.75)
  line L14 (-61.5877, 62.75) -> (-58.4123, 62.75)
  line L15 (-58.4123, 62.75) -> (-56.8246, 60)
  line L16 (56.8246, -60) -> (58.4123, -57.25)
  line L17 (58.4123, -57.25) -> (61.5877, -57.25)
  line L18 (61.5877, -57.25) -> (63.1754, -60)
  line L19 (63.1754, -60) -> (61.5877, -62.75)
  line L20 (61.5877, -62.75) -> (58.4123, -62.75)
  line L21 (58.4123, -62.75) -> (56.8246, -60)
  line L22 (63.1754, 60) -> (61.5877, 57.25)
  line L23 (61.5877, 57.25) -> (58.4123, 57.25)
  line L24 (58.4123, 57.25) -> (56.8246, 60)
  line L25 (56.8246, 60) -> (58.4123, 62.75)
  line L26 (58.4123, 62.75) -> (61.5877, 62.75)
  line L27 (61.5877, 62.75) -> (63.1754, 60)
  line L28 (-81.225, 54.775) -> (-81.225, 60.225)
  line L29 (-81.225, 60.225) -> (-75.775, 60.225)
  line L30 (-75.775, 60.225) -> (-75.775, 54.775)
  line L31 (-75.775, 54.775) -> (-81.225, 54.775)
  line L32 (-75.775, -54.775) -> (-75.775, -60.225)
  line L33 (-75.775, -60.225) -> (-81.225, -60.225)
  line L34 (-81.225, -60.225) -> (-81.225, -54.775)
  line L35 (-81.225, -54.775) -> (-75.775, -54.775)
  line L36 (81.225, 54.775) -> (75.775, 54.775)
  line L37 (75.775, 54.775) -> (75.775, 60.225)
  line L38 (75.775, 60.225) -> (81.225, 60.225)
  line L39 (81.225, 60.225) -> (81.225, 54.775)
  line L40 (81.225, -54.775) -> (81.225, -60.225)
  line L41 (81.225, -60.225) -> (75.775, -60.225)
  line L42 (75.775, -60.225) -> (75.775, -54.775)
  line L43 (75.775, -54.775) -> (81.225, -54.775)
  line L44 (82.75, -54) -> (-82.75, -54)
  arc A2 (-83.75, -53) -> (-82.75, -54) centre (-82.75, -53) ccw
  line L45 (-83.75, -53) -> (-83.75, 53)
  arc A3 (-82.75, 54) -> (-83.75, 53) centre (-82.75, 53) ccw
  line L46 (-82.75, 54) -> (82.75, 54)
  arc A4 (83.75, 53) -> (82.75, 54) centre (82.75, 53) ccw
  line L47 (83.75, 53) -> (83.75, -53)
  arc A5 (82.75, -54) -> (83.75, -53) centre (82.75, -53) ccw
  line L48 (89.5, 68) -> (-89.5, 68) construction
  line L49 (-89.5, 68) -> (89.5, 68) construction
  line L50 (-87, 65.4615) -> (-87, -61)
  arc A6 (-87, -61) -> (-86, -62) centre (-86, -61) ccw
  line L51 (-86, -62) -> (86, -62)
  arc A7 (86, -62) -> (87, -61) centre (86, -61) ccw
  line L52 (87, -61) -> (87, 65.4615)
  line L53 (-93, 65.4615) -> (-93, -61)
  arc A8 (-93, -61) -> (-86, -68) centre (-86, -61) ccw
  line L54 (-86, -68) -> (86, -68)
  arc A9 (86, -68) -> (93, -61) centre (86, -61) ccw
  line L55 (93, -61) -> (93, 65.4615)
  line L56 (-87, 65.4615) -> (-87, 68)
  line L57 (-87, 68) -> (-93, 68)
  line L58 (-93, 68) -> (-93, 65.4615)
  line L59 (87, 65.4615) -> (87, 68)
  line L60 (108.75, 54) -> (108.75, 4)
  line L61 (111.75, 68) -> (111.75, 1)
  line L62 (111.75, 1) -> (93, 1)
  line L63 (108.75, 4) -> (90, 4)
  line L64 (-90, 65.4615) -> (-90, 68)
  line L65 (88, 4) -> (90, 4) construction
  line L66 (90, 4) -> (88, 4) construction
  line L67 (87, 68) -> (111.75, 68)
  line L68 (90, 68) -> (90, 65.4615)
  line L69 (90, 54) -> (88, 54) construction
  line L70 (88, 54) -> (90, 54) construction
  line L71 (87, 54) -> (108.75, 54)
  dimension "d50" = -3
  dimension "d51" = 3
  dimension "d52" = 25
  dimension "d53" = 3
  dimension "d54" = 3
  constraint perpendicular L0 L56
  constraint perpendicular L1 L57
  constraint parallel L53 L58
  constraint collinear L49 L57
  constraint perpendicular L0 L59
  constraint perpendicular L3 L62
  constraint coincident L3 L63.end
  constraint perpendicular L3 L63
  constraint coincident L55 L62.end
  constraint coincident L1.start L64.start
  constraint coincident L57 L64.end
  constraint perpendicular L57 L64
  constraint collinear L63 L66
  constraint perpendicular L61 L67
  constraint collinear L49 L67
  constraint coincident L67 L68.start
  constraint collinear L3 L68
  constraint coincident L3.end L68.end
  constraint coincident L52 L71.start
  constraint coincident L60 L71.end
  constraint perpendicular L60 L71
  constraint collinear L69 L71
  measures "d52" distance of L47 L60
  measures "d53" distance of L62 L63
  measures "d54" distance of L60 L61
extrude "Extrude1'" add sketch "Sketch1 (2)" along normal blind 2 separate body contours E0 L0 L3 L52 L59 L71 | L3 L55 L60 L61 L62 L63 L67 L68 L71 | E0 L0 L59 L67 L68 | L3 L55 L63 L71 | L0 E1 L1 A0 L2 A1 L3 L7 L8 L9 L19 L20 L21 L50 A6 L51 A7 L52 L56 L71 | L1 A0 L2 A1 L3 L53 A8 L54 A9 L55 L57 L58 L63 L64 | L55 L60 L63 L71 | L0 E1 L56 L57 L64 | L19 L20 L21 L51 | L7 L8 L9 L51 makes body 2 in component "Top Cover"
extrude "Extrude2" add sketch "Sketch1 (2)" against normal up to surface (15 mm away) contours L3 L55 L60 L61 L62 L63 L67 L68 L71 | L1 A0 L2 A1 L3 L53 A8 L54 A9 L55 L57 L58 L63 L64 bodies 2 in component "Top Cover"
sketch "Sketch2" plane through (-108.75, 0, 0) normal (1, 0, 0) x (0, 1, 0) in component "Top Cover"
  line L0 (-54, -15) -> (-4, -15)
  line L1 (-4, -15) -> (-4, 0)
  line L2 (-4, 0) -> (-54, 0)
  line L3 (-54, -4.8) -> (-4, -4.8)
  line L4 (61, -5.8) -> (63, -5.8) construction
  line L5 (61, -5.8) -> (63, -5.8) construction
  line L6 (61, -5.8) -> (56, -5.8) construction
  line L7 (54, -5.8) -> (56, -5.8) construction
  line L8 (53, -5.8) -> (54, -5.8) construction
  line L9 (59.15, -5.8) -> (55.85, -5.8) construction
  line L10 (-54, 0) -> (-54, -15)
  line L11 (-9.5, -4.8) -> (-18.5, -4.8) construction
  line L12 (-18.5, -4.8) -> (-9.5, -4.8) construction
  point P0 (-8.5, -5.8)
  point P1 (-4, -5.8)
  point P2 (-54, -5.8)
  point P3 (-19.5, -5.8)
  point P4 (-63, -5.8)
  constraint coincident L1 L3.end
  constraint perpendicular L1 L3
  constraint coincident L3.start L10
  constraint collinear L3 L11
extrude "Extrude3'" cut sketch "Sketch2" against normal up to surface (3 mm away) contours L0 L1 L3 L10 bodies 2 in component "Top Cover"
sketch "Sketch3 (2)" plane through (0, 0, 0) normal (0, 0, -1) x (1, 0, 0) in component "Top Cover"
  line L0 (-108.75, 54) -> (-108.75, 4)
  line L1 (-108.75, 4) -> (-90, 4)
  line L2 (-90, 68) -> (-90, 54)
  arc A0 (-90, -61) -> (-86, -65) centre (-86, -61) ccw
  line L3 (-86, -65) -> (86, -65)
  arc A1 (86, -65) -> (90, -61) centre (86, -61) ccw
  line L4 (90, -61) -> (90, 68)
  line L5 (90, 68) -> (87, 68)
  line L6 (87, 68) -> (87, -61)
  arc A2 (86, -62) -> (87, -61) centre (86, -61) ccw
  line L7 (86, -62) -> (-86, -62)
  arc A3 (-87, -61) -> (-86, -62) centre (-86, -61) ccw
  line L8 (-87, -61) -> (-87, 68)
  line L9 (-87, 68) -> (-90, 68)
  line L10 (-90, 68) -> (-90, 65)
  line L11 (-90, 54) -> (-108.75, 54)
  line L12 (-90, 4) -> (-90, -61)
  constraint coincident L2.start L9.end
extrude "Extrude4'" cut sketch "Sketch3 (2)" against normal blind 0.2 bodies 2 in component "Top Cover"
move_face "OffsetFaces1" offset -0.1 5 faces at (-90, 39.3333, -4.8667) (-86.757, 64.9277, -9.9333) (28.6667, 65, -4.8667) (88.8949, 63.7603, -4.8667) (90, -25, -9.9333) on bodies 2 in component "Top Cover"
sketch "Sketch4 (2)" plane through (93, 0, 0) normal (1, 0, 0) x (0, 1, 0) in component "Top Cover"
  line L0 (61, -15) -> (61, 2)
  line L1 (61, 2) -> (-68, 2)
  line L2 (-68, 2) -> (-68, -15)
  line L3 (-68, -15) -> (61, -15)
  circle A0 centre (-30, -3) radius 1.425 construction
  circle A1 centre (30, -3) radius 1.425 construction
  circle A2 centre (-30, -3) radius 1.65
  circle A3 centre (30, -3) radius 1.65
  dimension "d74" = 3.3
  constraint concentric A0 A2
  constraint concentric A1 A3
  constraint equal A2 A3
  measures "d74" diameter of A2
extrude "Extrude5'" cut sketch "Sketch4 (2)" against normal up to surface (204.75 mm away) contours A2 | A3 bodies 2 in component "Top Cover"
sketch "Sketch5 (2)" plane through (0, 68, 0) normal (0, 1, 0) x (-1, 0, 0) in component "Top Cover"
  line L0 (86, -15) -> (86, 2)
  line L1 (86, 2) -> (-86, 2)
  line L2 (-86, 2) -> (-86, -15)
  line L3 (-86, -15) -> (86, -15)
  circle A0 centre (-70, -4) radius 1.425 construction
  circle A1 centre (0, -4) radius 1.425 construction
  circle A2 centre (70, -4) radius 1.425 construction
  circle A3 centre (70, -4) radius 1.5
  circle A4 centre (0, -4) radius 1.5
  circle A5 centre (-70, -4) radius 1.5
  dimension "d75" = 3
  constraint concentric A2 A3
  constraint concentric A1 A4
  constraint concentric A0 A5
  constraint equal A4 A5
  constraint equal A3 A4
  measures "d75" diameter of A3
extrude "Extrude6'" cut sketch "Sketch5 (2)" against normal up to surface (2.9 mm away) contours A3 | A4 | A5 bodies 2 in component "Top Cover"
fillet "Fillet1" radius 1 4 edges at (93, -68, -6.5) (-111.75, -68, -6.5) (-87, -68, 1.1) (87, -68, 1.1) on bodies 2 in component "Top Cover"
fillet "Fillet2" radius 2 2 edges at (-93, -1, -6.5) (-111.75, -1, -6.5) on bodies 2 in component "Top Cover"
fillet "Fillet3" radius 0.5 20 edges at (-87.2929, -67.7071, 2) (-87, -3, 2) (-86.7071, 61.7071, 2) (0, 62, 2) (86.7071, 61.7071, 2) (87, -3, 2) (87.2929, -67.7071, 2) (90, -68, 2) (92.7071, -67.7071, 2) (93, -3, 2) (90.9497, 65.9497, 2) (0, 68, 2) (-90.9497, 65.9497, 2) (-93, 31, 2) (-93.5858, -0.4142, 2) (-102.375, -1, 2) (-111.1642, -1.5858, 2) (-111.75, -35, 2) (-111.4571, -67.7071, 2) (-99.375, -68, 2) on bodies 2 in component "Top Cover"
fillet "Fillet4" radius 0.5 6 edges at (-90.1, -4, -7.4) (-90, -54, -7.4) (90.1, -68, -7.4) (-90, -68, -7.4) (-111.75, -4, -9.9) (-111.75, -54, -9.9) on bodies 2 in component "Top Cover"